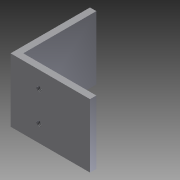
# Autodesk Inventor part: 13_0204_070
Saved by Autodesk Inventor 2012 SP1 (Build 160190100, 190)
## iProperties
Created: 2013-05-07
Part Number: 13_0204_070
Material: Default
Document SubType Name: Modeling
Designer: vogel
Density: 1 g/cm^3
Author: vogel
Autodesk Inventor part; units mm, degrees
ref_plane "YZ Plane" through (0, 0, 0) normal (1, 0, 0) x (0, 1, 0)
ref_plane "XZ Plane" through (0, 0, 0) normal (0, 1, 0) x (-1, 0, 0)
ref_plane "XY Plane" through (0, 0, 0) normal (0, 0, 1) x (1, 0, 0)
sketch "Skizze1" plane through (0, 0, 0) normal (0, 0, 1) x (1, 0, 0)
  line L0 (0, 0) -> (25, 0)
  line L1 (2, 2) -> (2, 25)
  line L2 (2, 25) -> (0, 25)
  line L3 (0, 25) -> (0, 0)
  line L4 (2, 2) -> (25, 2)
  line L5 (25, 2) -> (25, 0)
  dimension "d0" = 2
  dimension "d1" = 25
  dimension "d2" = 25
  constraints: 12 end point, 4 perpendicular, 2 parallel, 1 horizontal
  measures "d0" distance between parallel lines of L3 L1
  measures "d1" distance between parallel lines of L2 L0
  measures "d2" distance of L0.start L0.end
extrude "Extrusion1" add sketch "Skizze1" along normal blind 20
sketch "Skizze2" plane through (0, 0, 0) normal (0, -1, 0) x (1, 0, 0)
  line L0 (25, 20) -> (0, 20) projected
  line L1 (0, 0) -> (0, 20) projected
  line L2 (0, 0) -> (25, 0) projected
  line L3 (25, 0) -> (25, 20) projected
  line L4 (9, 20) -> (9, 0)
  line L5 (0, 10) -> (25, 10)
  point P0 (9, 14.7)
  point P1 (9, 5.3)
  dimension "d5" = 9
  dimension "d6" = 9.4
  constraints: 4 end point, 4 point on line, 2 midpoint, 1 perpendicular, 1 symmetric about line
  measures "d5" distance between parallel lines of L4 L1
  measures "d6" distance of point (9, 14.7) point (9, 5.3)
hole "Bohrung1" at (9, 0, 14.7) at (9, 0, 5.3) direction (0, 1, 0) diameter 1.567 end through all thread size "M2x0.4" class "6H" standard "ISO Metric profile"
sketch "Skizze3" plane through (2, 2, 0) normal (1, 0, 0) x (0, 0, -1)
  line L0 (0, 0) -> (-20, 0) projected
  line L1 (0, 23) -> (-20, 23) projected
  line L2 (-13.3, 20) -> (-13.3, 10)
  line L3 (-16.7, 10) -> (-16.7, 20)
  line L4 (-3.3, 20) -> (-3.3, 10)
  line L5 (-6.7, 10) -> (-6.7, 20)
  line L6 (-10, 23) -> (-10, 0)
  line L7 (-15, 20) -> (-15, 10)
  line L8 (-5, 10) -> (-5, 20)
  arc A0 (-13.3, 20) -> (-16.7, 20) centre (-15, 20) ccw
  arc A1 (-3.3, 20) -> (-6.7, 20) centre (-5, 20) ccw
  arc A2 (-6.7, 10) -> (-3.3, 10) centre (-5, 10) ccw
  arc A3 (-16.7, 10) -> (-13.3, 10) centre (-15, 10) ccw
  point P0 (0, -2)
  dimension "d14" = 10
  dimension "d15" = 3.4
  dimension "d16" = 3
  dimension "d18" = 10
  constraints: 14 end point, 8 point on circle, 8 tangent, 4 centre point, 4 coincident, 3 parallel, 2 midpoint, 1 horizontal alignment, 4 other
  measures "d14" distance between parallel lines of L8 L7
  measures "d15" distance between parallel lines of L3 L2
  measures "d16" distance from line of L1 A0.centre
  measures "d18" distance of L3.start L3.end
extrude "Extrusion2" cut sketch "Skizze3" against normal through all
